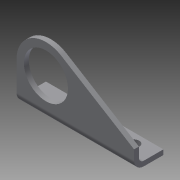
# Autodesk Inventor part: Flange Bearing Mount Tower Mirror
Saved by Autodesk Inventor 2013 (Build 170138000, 138)
## iProperties
Created: 2013-01-21
Part Number: Flange Bearing Mount Tower Mirror
Material: Generic
Document SubType Name: Sheet Metal
Designer: actoennies
Density: 1 g/cm^3
Sheet Metal Rule: Default
Mass: 8.97134 g
Surface Area: 68.258 cm^2
Volume: 8.97134 cm^3
Author: actoennies
Autodesk Inventor part; units mm, degrees
ref_plane "YZ Plane" through (0, 0, 0) normal (1, 0, 0) x (0, 1, 0)
ref_plane "XZ Plane" through (0, 0, 0) normal (0, 1, 0) x (-1, 0, 0)
ref_plane "XY Plane" through (0, 0, 0) normal (0, 0, 1) x (1, 0, 0)
sketch "Sketch1" plane through (0, 0, 0) normal (0, 1, 0) x (-1, 0, 0)
  line L0 (0, 0) -> (-76.2, 0)
  line L1 (-76.2, 0) -> (-76.2, 12.7)
  line L2 (-76.2, 12.7) -> (-38.1, 12.7)
  line L3 (0, 12.7) -> (0, 0)
  line L4 (0, 0) -> (-12.7, 0)
  circle A0 centre (-38.1, 6.35) radius 3.3782
  circle A1 centre (-63.5, 6.35) radius 3.3782
  line L5 (-38.1, 12.7) -> (0, 12.7)
  dimension "d0" = 12.7
  dimension "d1" = 76.2
  dimension "d2" = 6.7564
  dimension "d3" = 6.7564
  dimension "d4" = 6.35
  dimension "d5" = 38.1
  dimension "d6" = 6.35
  dimension "d7" = 12.7
  dimension "d8" = 38.1
  measures "d0" distance between parallel lines of L0 L2
  measures "d1" distance of L1.end L3.start
  measures "d2" diameter of A0
  measures "d3" diameter of A1
  measures "d4" distance from line of L0 A0.centre
  measures "d5" distance from line of L3 A0.centre
  measures "d6" distance from line of L2 A1.centre
  measures "d7" distance from line of L1 A1.centre
  measures "d8" distance of L1.end L2.end
extrude "Plate1" add sketch "Sketch1" along normal blind 3.175
sketch "Sketch2" plane through (76.2, 6.35, 15.875) normal (0, 0, 1) x (1, 0, 0)
  line L0 (-76.2, 0) -> (0, 0)
  line L1 (0, 0) -> (0, 38.1)
  line L2 (0, 38.1) -> (-76.2, 38.1)
  line L3 (-76.2, 38.1) -> (-76.2, 0)
  constraints: 6 end point, 1 horizontal, 1 perpendicular, 1 vertical
edge flange "Flange1" height 44.45 angle 90 thickness 3.175 bend radius 3.175 thickness toward (0, 0, 1) relief straight relief width 3.175 relief depth 1.5875 corner gap 3.175 corner form 0 edges at (19.05, 3.175, 12.7) (57.15, 3.175, 12.7) wall of the first edge with corners at (0, 6.35, 15.875) (76.2, 6.35, 15.875) (76.2, 44.45, 15.875) (0, 44.45, 15.875)
bend "Bend1"
corner "Corner1"
sketch "Sketch3" plane through (76.2, 44.45, 15.875) normal (0, 0, -1) x (-1, 0, 0)
  line L0 (0, -38.1) -> (76.2, -38.1) projected
  line L1 (76.2, 0) -> (76.2, -38.1) projected
  line L2 (76.2, 0) -> (0, 0) projected
  line L3 (0, 0) -> (0, -38.1) projected
  circle A0 centre (57.15, -19.05) radius 14.2875
  arc A1 (76.2, -19.05) -> (47.1912, -2.8104) centre (57.15, -19.05) ccw
  line L4 (0, -31.75) -> (47.1912, -2.8104)
  point P0 (76.2, -44.45)
  dimension "d20" = 28.575
  dimension "d21" = 19.05
  dimension "d22" = 19.05
  dimension "d23" = 6.35
  constraints: 2 centre point, 2 end point, 2 point on circle, 2 tangent, 1 coincident, 1 midpoint, 1 point on line
  measures "d20" diameter of A0
  measures "d21" distance from line of L1 A0.centre
  measures "d22" distance from line of L2 A0.centre
  measures "d23" distance from line of L0 L4.start
extrude "Cut1" cut sketch "Sketch3" against normal blind 3.175 contours L3 L2 A1 L4 | A1 L2 L1 | A0
equation "\"d24\" = Thickness"
equation "\"d10\" = BendReliefWidth"
equation "\"d11\" = BendReliefDepth"
equation "\"d12\" = MinimumRemnant"
equation "\"d13\" = BendRadius"
equation "\"d16\" = BendRadius"
equation "\"d17\" = CornerReliefSize"
equation "\"d18\" = GapSize"
equation "\"d19\" = JacobiRadiusSize"
equation "\"BendRadius\" = Thickness"
equation "\"BendReliefWidth\" = Thickness"
equation "\"BendReliefDepth\" = 0.5 * Thickness"
equation "\"CornerReliefSize\" = 4 * Thickness"
equation "\"MinimumRemnant\" = 2 * Thickness"
equation "\"TransitionRadius\" = BendRadius"
equation "\"JacobiRadiusSize\" = BendRadius"
equation "\"GapSize\" = Thickness"
equation "\"d9\" = BendRadius"
equation "\"Thickness\" = 3.175"
body "Solid1"
